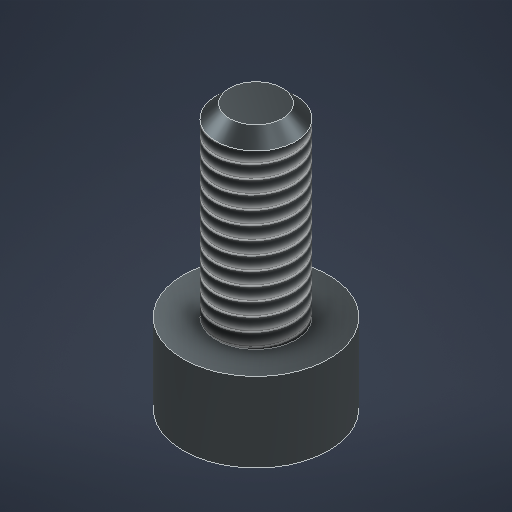
# Autodesk Inventor part: TornilloM3
Saved by Autodesk Inventor 2026.1 (Build 301233000, 233)
## iProperties
Created: 2025-12-08
Part Number: TornilloM3
Material: Hierro, gris
Document SubType Name: Modeling
Designer: vickh
Density: 7.15 g/cm^3
Appearance: Gris hierro
Author: vickh
Autodesk Inventor part; units mm, degrees
ref_plane "YZ Plane" through (0, 0, 0) normal (1, 0, 0) x (0, 1, 0)
ref_plane "XZ Plane" through (0, 0, 0) normal (0, 1, 0) x (-1, 0, 0)
ref_plane "XY Plane" through (0, 0, 0) normal (0, 0, 1) x (1, 0, 0)
sketch "Boceto1" plane through (0, 0, 0) normal (0, 1, 0) x (-1, 0, 0)
  circle A0 centre (0, 0) radius 2.75
  dimension "d0" = 5.5
  constraints: 1 centre point, 1 coincident
  measures "d0" diameter of A0
extrude "Extrusión1" add sketch "Boceto1" along normal blind 3
sketch "Boceto2" plane through (0, 0, 0) normal (0, -1, 0) x (1, 0, 0)
  point P0 (0, 0)
  point P1 (0, 0)
  constraints: 1 coincident
hole "Agujero1" at (0, 0, 0) direction (0, 1, 0) diameter 2.58 depth 1.3 tip angle 118
sketch "Boceto3" plane through (0, 0, 0) normal (0, -1, 0) x (1, 0, 0)
  circle A0 centre (0, 0) radius 1.29 projected
  line L0 (0, 1.4896) -> (1.29, 0.7448)
  line L1 (1.29, 0.7448) -> (1.29, -0.7448)
  line L2 (1.29, -0.7448) -> (0, -1.4896)
  line L3 (0, -1.4896) -> (-1.29, -0.7448)
  line L4 (-1.29, -0.7448) -> (-1.29, 0.7448)
  line L5 (-1.29, 0.7448) -> (0, 1.4896)
  constraints: 12 end point, 1 coincident, 1 tangent, 1 vertical, 13 other
extrude "Extrusión2" cut sketch "Boceto3" against normal blind 1.3
sketch "Boceto4" plane through (0, 3, 0) normal (0, 1, 0) x (1, 0, 0)
  circle A0 centre (0, 0) radius 1.5
  dimension "d12" = 3
  constraints: 1 centre point, 1 coincident
  measures "d12" diameter of A0
extrude "Extrusión3" add sketch "Boceto4" along normal blind 7
thread "Rosca1" size "M3x0.5" class "6g" standard "ANSI Metric M Profile" full length
chamfer "Chaflán1" distance 0.5 angle 45 1 edges at (-1.5, 10, 0)
